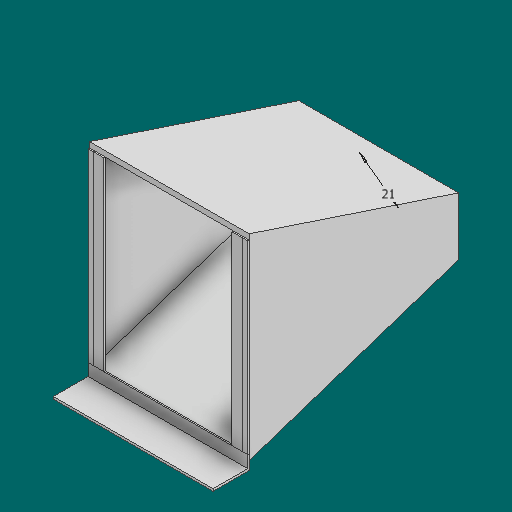
# Autodesk Inventor part: CamBody
Saved by Autodesk Inventor 2025.2 (Build 292293000, 293)
## iProperties
Created: 2025-04-19
Part Number: CamBody
Material: Generic
Document SubType Name: Modeling
Designer: Matt Caldwell
Density: 1 g/cm^3
Appearance: Default
Author: Matt Caldwell
Autodesk Inventor part; units mm, degrees
ref_plane "Work Plane1" through (0, 32.027, -88.9) normal (0, 0, -1) x (-1, 0, 0)
ref_plane "Work Plane2" through (62.86, 0, 0) normal (1, 0, 0) x (0, 0, -1)
ref_plane "Work Plane4" through (65.86, 0, 0) normal (1, 0, 0) x (0, 0, -1)
sketch "Sketch14" plane through (65.86, 0, 0) normal (1, 0, 0) x (0, 0, -1)
  line L0 (0, 0) -> (0, 80) projected
  line L1 (0, 0) -> (0, -2.5)
  line L2 (0, -2.5) -> (90.4875, 27.4259)
  line L3 (90.4875, 27.4259) -> (90.4875, 52.4259)
  line L4 (90.4875, 52.4259) -> (0, 82.3518)
  line L5 (0, 82.3518) -> (0, 80)
  line L6 (0, 80) -> (87.3125, 51.1242)
  line L7 (87.5, 51.0621) -> (87.5, 28.9379) projected
  line L8 (87.3125, 51.1242) -> (87.5, 51.0621)
  line L9 (87.5, 51.0621) -> (87.5, 28.9379)
  line L10 (87.5, 28.9379) -> (0, 0)
  dimension "d60" = 2.5
  dimension "d61" = 71.7
  dimension "d62" = 25
  dimension "d63" = 108.3
  constraints: 18 end point, 2 collinear, 2 parallel, 1 point on line, 1 vertical
  measures "d60" distance of L0.start L1.end
  measures "d61" angle of L2 L1
  measures "d62" distance of L2.end L3.end
  measures "d63" angle of L4 L3
extrude "Extrusion10" add sketch "Sketch14" against normal blind 64 contours L10 L7 L8 L6 L5 L4 L3 L2 L1
ref_plane "Work Plane5" through (1.86, 0, 0) normal (-1, 0, 0) x (0, 0, 1)
sketch "Sketch15" plane through (1.86, 0, 0) normal (-1, 0, 0) x (0, 0, 1)
  line L0 (0, 82.3518) -> (-90.4875, 52.4259) projected
  line L1 (0, 82.3518) -> (-90.4875, 52.4259)
  line L2 (-90.4875, 52.4259) -> (-90.4875, 27.4259) projected
  line L3 (-90.4875, 52.4259) -> (-90.4875, 27.4259)
  line L4 (0, -2.5) -> (-90.4875, 27.4259) projected
  line L5 (-90.4875, 27.4259) -> (0, -2.5)
  line L6 (0, -2.5) -> (0, 82.3518)
  point P0 (0, 0)
  constraints: 8 end point, 3 collinear, 1 parallel
extrude "Extrusion11" add sketch "Sketch15" along normal blind 2.5
sketch "Sketch16" plane through (65.86, 0, 0) normal (1, 0, 0) x (0, 0, -1)
  line L0 (90.4875, 52.4259) -> (0, 82.3518) projected
  line L1 (90.4875, 27.4259) -> (90.4875, 52.4259) projected
  line L2 (0, 82.3518) -> (90.4875, 52.4259)
  line L3 (90.4875, 52.4259) -> (90.4875, 27.4259)
  line L4 (0, -2.5) -> (90.4875, 27.4259) projected
  line L5 (90.4875, 27.4259) -> (0, -2.5)
  line L6 (0, 82.3518) -> (0, 80) projected
  line L7 (0, -2.5) -> (0, 82.3518)
  point P0 (0, 0)
  constraints: 8 end point, 3 collinear
extrude "Extrusion12" add sketch "Sketch16" along normal blind 2.5
sketch "Sketch17" plane through (-0.64, -2.5, 0) normal (0, 0, 1) x (1, 0, 0)
  line L0 (2.5, 2.5) -> (2.5, 82.5) projected
  line L1 (0, 0) -> (0, 84.8518) projected
  line L2 (2.5, 82.5) -> (0, 82.5)
  line L3 (0, 82.5) -> (0, 2.5)
  line L4 (0, 2.5) -> (2.5, 2.5)
  line L5 (2.5, 2.5) -> (2.5, 82.5)
  line L6 (66.5, 82.5) -> (66.5, 2.5) projected
  line L7 (69, 84.8518) -> (69, 0) projected
  line L8 (66.5, 82.5) -> (69, 82.5)
  line L9 (69, 82.5) -> (69, 2.5)
  line L10 (69, 2.5) -> (66.5, 2.5)
  line L11 (66.5, 2.5) -> (66.5, 82.5)
  point P0 (0.64, 2.5)
  constraints: 16 end point, 4 parallel, 3 point on line, 2 horizontal, 2 perpendicular
extrude "Extrusion13" add sketch "Sketch17" along normal blind 0.6 separate body
sketch "Sketch18" plane through (65.86, 0, 0) normal (-1, 0, 0) x (0, 0, 1)
  line L0 (0.6, 0) -> (0.6, 80) projected
  line L1 (0, 80) -> (0.6, 80)
  line L2 (0.6, 80) -> (0.6, 0)
  line L3 (0.6, 0) -> (0, 0)
  line L4 (0, 0) -> (0, 80)
  constraints: 8 end point, 2 parallel, 1 horizontal, 1 perpendicular
extrude "Extrusion14" add sketch "Sketch18" along normal blind 4.35 separate body
sketch "Sketch19" plane through (1.86, 0, 0) normal (1, 0, 0) x (0, 0, -1)
  line L0 (-0.6, 80) -> (0, 80)
  line L1 (0, 80) -> (0, 0)
  line L2 (0, 0) -> (-0.6, 0)
  line L3 (-0.6, 0) -> (-0.6, 80)
  constraints: 8 end point, 2 parallel, 1 horizontal, 1 perpendicular
extrude "Extrusion15" add sketch "Sketch19" along normal blind 4.35 separate body
sketch "Sketch25" plane through (-0.64, -2.5, 0) normal (0, 0, 1) x (1, 0, 0)
  line L0 (66.5, 2.5) -> (69, 2.5) projected
  line L1 (69, 2.5) -> (0, 2.5)
  line L2 (0, 2.5) -> (0, -2.7)
  line L3 (0, -2.7) -> (69, -2.7)
  line L4 (69, -2.7) -> (69, 2.5)
  point P0 (0.64, 2.5)
  dimension "d106" = 5.2
  constraints: 8 end point, 2 parallel, 1 horizontal, 1 perpendicular
  measures "d106" distance of L2.end L1.end
extrude "Extrusion17" add sketch "Sketch25" along normal blind 0.6 separate body
sketch "Sketch26" plane through (-0.64, -2.5, 0.6) normal (0, 0, 1) x (1, 0, 0)
  line L0 (0, 2.5) -> (0, -2.7) projected
  line L1 (0, -2.7) -> (69, -2.7)
  line L2 (69, -2.7) -> (69, -3.7)
  line L3 (69, -3.7) -> (0, -3.7)
  line L4 (0, -3.7) -> (0, -2.7)
  point P0 (0.64, 2.5)
  dimension "d109" = 1
  constraints: 8 end point, 2 parallel, 1 horizontal, 1 perpendicular
  measures "d109" distance of L1.end L2.end
extrude "Extrusion18" add sketch "Sketch26" along normal blind 15 bodies 5
sketch "Sketch27" plane through (-0.64, -2.5, 0.6) normal (0, 0, -1) x (-1, 0, 0)
  line L0 (-69, -3.7) -> (-69, -2.7) projected
  line L1 (0, -2.7) -> (-69, -2.7) projected
  line L2 (-69, -3.7) -> (0, -3.7)
  line L3 (0, -3.7) -> (0, -2.7)
  line L4 (0, -2.7) -> (-69, -2.7)
  line L5 (-69, -2.7) -> (-69, -3.7)
  point P0 (-0.64, 2.5)
  constraints: 8 end point, 2 parallel, 1 horizontal, 1 perpendicular
extrude "Extrusion19" add sketch "Sketch27" along normal blind 0.6 bodies 5
sketch "Sketch28" plane through (-0.64, 27.4259, -90.4875) normal (0, 0, -1) x (-1, 0, 0)
  circle A0 centre (-34.474, 12.5607) radius 10.5
  point P0 (-0.64, -27.4259)
  dimension "d114" = 21
  constraints: 1 centre point
  measures "d114" diameter of A0
body "Solid2"
body "Solid7"
body "Solid8"
body "Solid9"
body "Solid10"
body "Solid12"
